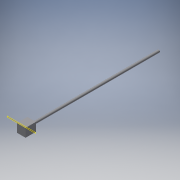
# Autodesk Inventor part: MotorandLeadscrew
Saved by Autodesk Inventor 2016 (Build 200138000, 138)
## iProperties
Created: 2016-05-26
Part Number: MotorandLeadscrew
Material: Generic
Document SubType Name: Modeling
Designer: Scott
Density: 1 g/cm^3
Appearance: Default
Author: Scott
Autodesk Inventor part; units mm, degrees
ref_plane "YZ Plane" through (0, 0, 0) normal (1, 0, 0) x (0, 1, 0)
ref_plane "XZ Plane" through (0, 0, 0) normal (0, 1, 0) x (-1, 0, 0)
ref_plane "XY Plane" through (0, 0, 0) normal (0, 0, 1) x (1, 0, 0)
ref_plane "Work Plane1" through (-337.8481, -441.0413, 0) normal (0, 0, 1) x (1, 0, 0)
sketch "Sketch1" plane through (-337.8481, -441.0413, 0) normal (0, 0, 1) x (1, 0, 0)
  line L0 (-84.5, -47.3468) -> (-42.5, -47.3468)
  line L1 (-42.5, -47.3468) -> (-42.5, -5.3468)
  line L2 (-42.5, -5.3468) -> (-84.5, -5.3468)
  line L3 (-84.5, -5.3468) -> (-84.5, -47.3468)
  line L4 (-84.5, -47.3468) -> (-42.5, -5.3468) construction
  line L5 (-42.5, -47.3468) -> (-84.5, -5.3468) construction
  point P0 (337.8481, 441.0413)
  point P1 (-63.5, -26.3468)
  dimension "d0" = 42
  dimension "d1" = 42
  constraints: 12 end point, 2 midpoint, 2 parallel, 1 horizontal, 1 perpendicular
  measures "d0" distance of L2.end L1.end
  measures "d1" distance of L1.end L0.end
extrude "Extrusion1" add sketch "Sketch1" against normal blind 50.8
sketch "Sketch2" plane through (-337.8481, -441.0413, -50.8) normal (0, 0, -1) x (-1, 0, 0)
  line L0 (42.5, -47.3468) -> (84.5, -47.3468) projected
  line L1 (84.5, -47.3468) -> (84.5, -5.3468) projected
  line L2 (84.5, -5.3468) -> (42.5, -5.3468) projected
  line L3 (42.5, -5.3468) -> (42.5, -47.3468) projected
  circle A0 centre (63.5, -26.3468) radius 6.35
  point P0 (-337.8481, 441.0413)
  dimension "d4" = 12.7
  constraints: 1 centre point
  measures "d4" diameter of A0
extrude "Extrusion2" add sketch "Sketch2" along normal blind 622.3 contours A0
sketch "Sketch3" plane through (-337.8481, -441.0413, -50.8) normal (0, 0, -1) x (-1, 0, 0)
  circle A0 centre (63.5, -26.3468) radius 6.35 projected
  line L0 (42.5, -47.3468) -> (84.5, -47.3468) projected
  line L1 (84.5, -47.3468) -> (84.5, -5.3468) projected
  line L2 (84.5, -5.3468) -> (42.5, -5.3468) projected
  line L3 (42.5, -5.3468) -> (42.5, -47.3468) projected
  circle A1 centre (63.5, -26.3468) radius 19.05
  point P0 (-337.8481, 441.0413)
  dimension "d7" = 38.1
  constraints: 1 centre point, 1 coincident
  measures "d7" diameter of A1
extrude "Extrusion3" add sketch "Sketch3" along normal blind 38.1 contours A1
sketch "Sketch4" plane through (-337.8481, -441.0413, -50.8) normal (0, 0, -1) x (-1, 0, 0)
  circle A0 centre (63.5, -26.3468) radius 19.05 projected
  line L0 (42.5, -47.3468) -> (84.5, -47.3468) projected
  line L1 (84.5, -47.3468) -> (84.5, -5.3468) projected
  line L2 (84.5, -5.3468) -> (42.5, -5.3468) projected
  line L3 (42.5, -5.3468) -> (42.5, -47.3468) projected
  circle A1 centre (63.5, -26.3468) radius 6.35 projected
  point P0 (-337.8481, 441.0413)
extrude "Extrusion4" cut sketch "Sketch4" along normal mid plane 5.08 contours A0 | L3 L2 L1 L0
body "Solid1"
